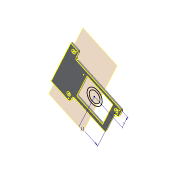
# Autodesk Inventor part: 00_KES400_Bluray_Lens
Saved by Autodesk Inventor 2019 (Build 230136000, 136)
## iProperties
Created: 2018-10-09
Part Number: 00_KES400_Bluray_Lens
Material: Generic
Document SubType Name: Modeling
Designer: diederichbenedict
Density: 1 g/cm^3
Appearance: Default
Author: diederichbenedict
Autodesk Inventor part; units mm, degrees
ref_plane "YZ Plane" through (0, 0, 0) normal (1, 0, 0) x (0, 1, 0)
ref_plane "XZ Plane" through (0, 0, 0) normal (0, 1, 0) x (-1, 0, 0)
ref_plane "XY Plane" through (0, 0, 0) normal (0, 0, 1) x (1, 0, 0)
ref_plane "Work Plane1" through (7.2162, 6.7561, 0) normal (0, 0, 1) x (-0.4175, -0.9087, 0)
sketch "Sketch1" plane through (7.2162, 6.7561, 0) normal (0, 0, 1) x (-0.4175, -0.9087, 0)
  circle A0 centre (9.5108, 16.1864) radius 1
  circle A1 centre (25.0108, -5.3136) radius 1
  circle A2 centre (4.5108, -11.8136) radius 1
  line L0 (22.0108, -1.8136) -> (8.5108, -1.8136)
  line L1 (8.5108, -1.8136) -> (8.5108, 13.6864)
  line L2 (8.5108, 13.6864) -> (22.0108, 13.6864)
  line L3 (22.0108, 13.6864) -> (22.0108, -1.8136)
  line L4 (11.1138, 15.6864) -> (23.6484, 15.6864)
  line L5 (23.6484, 15.6864) -> (23.6484, -3.7858)
  line L6 (23.6484, -3.7858) -> (27.5108, -3.7858)
  line L7 (27.5108, -3.7858) -> (27.5108, -8.9631)
  line L8 (27.5108, -8.9631) -> (27.5108, -14.3136)
  line L9 (27.5108, -14.3136) -> (1.8108, -14.3136)
  line L10 (1.8108, -14.3136) -> (1.8108, -10.169)
  line L11 (1.8108, -10.169) -> (6.5484, -10.169)
  line L12 (6.5484, -10.169) -> (6.5484, 18.6864)
  line L13 (6.5484, 18.6864) -> (11.1138, 18.6864)
  line L14 (11.1138, 18.6864) -> (11.1138, 15.6864)
  point P0 (9.1519, -3.7364)
  dimension "d0" = 2
  dimension "d1" = 2
  dimension "d2" = 2
  dimension "d3" = 28
  dimension "d5" = 15.5
  dimension "d6" = 5
  dimension "d8" = 20.5
  dimension "d9" = 2.5
  dimension "d10" = 1
  dimension "d12" = 3
  dimension "d13" = 33
  dimension "d14" = 25.7
  dimension "d15" = 17.1
  dimension "d23" = 30.5
  dimension "d24" = 9
  dimension "d25" = 2.5
  constraints: 30 end point, 10 perpendicular, 3 centre point, 2 horizontal, 2 parallel, 1 point on line
  measures "d0" diameter of A0
  measures "d1" diameter of A1
  measures "d2" diameter of A2
  measures "d3" vertical distance of A0.centre A2.centre
  measures "d5" horizontal distance of A0.centre A1.centre
  measures "d6" horizontal distance of A2.centre A0.centre
  measures "d8" horizontal distance of A2.centre A1.centre
  measures "d9" distance from line of A0.centre L2
  measures "d10" distance from line of L1 A0.centre
  measures "d12" distance from line of A1.centre L3
  measures "d13" distance between parallel lines of L13 L9
  measures "d14" distance between parallel lines of L10 L7
  measures "d15" distance between parallel lines of L5 L12
  measures "d23" distance from line of L9 A0.centre
  measures "d24" distance from line of A1.centre L9
  measures "d25" distance from line of A1.centre L8
extrude "Extrusion1" add sketch "Sketch1" along normal blind 1
fillet "Fillet1" radius 1 7 edges at (21.4621, -6.996, 0.5) (19.556, -11.1444, 0.5) (16.83, -9.8919, 0.5) (-6.0973, -13.1521, 0.5) (-7.7098, -16.6617, 0.5) (-2.7802, 9.3562, 0.5) (-4.7582, 5.0513, 0.5)
body "Solid1"
